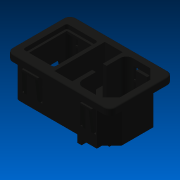
# Autodesk Inventor part: Soanar Power Module Housing
Saved by Autodesk Inventor 2016 (Build 200138000, 138)
## iProperties
Created: 2013-08-06
Material: ABS Plastic
Document SubType Name: Modeling
Designer: sdarley
Density: 1.06 g/cm^3
Appearance: Smooth - Black
Project: Power Entry Module - Soanar PP4003
Description: Soanar Power Module Housing
Author: sdarley
Title: Soanar Power Module Housing
Revision Number: 1
Autodesk Inventor part; units mm, degrees
ref_plane "YZ Plane" through (0, 0, 0) normal (1, 0, 0) x (0, 1, 0)
sketch "Sketch1" plane through (0, 0, 0) normal (0, 1, 0) x (-1, 0, 0)
  line L0 (-22, -15.3) -> (22, -15.3)
  line L1 (25, -12.3) -> (25, 12.3)
  line L2 (22, 15.3) -> (-22, 15.3)
  line L3 (-25, 12.3) -> (-25, -12.3)
  line L4 (-25, -15.3) -> (25, 15.3) construction
  line L5 (25, -15.3) -> (-25, 15.3) construction
  arc A0 (-22, 15.3) -> (-25, 12.3) centre (-22, 12.3) ccw
  arc A1 (-25, -12.3) -> (-22, -15.3) centre (-22, -12.3) ccw
  arc A2 (22, -15.3) -> (25, -12.3) centre (22, -12.3) ccw
  arc A3 (25, 12.3) -> (22, 15.3) centre (22, 12.3) ccw
  line L6 (20.8, 10.65) -> (7.8, 10.65)
  line L7 (6.8, 9.65) -> (6.8, -9.65)
  line L8 (7.8, -10.65) -> (20.8, -10.65)
  line L9 (21.8, -9.65) -> (21.8, 9.65)
  line L10 (5, 12.15) -> (-3.6, 12.15)
  line L11 (-3.6, -12.15) -> (5, -12.15)
  line L12 (5, -12.15) -> (5, 12.15)
  arc A4 (7.8, 10.65) -> (6.8, 9.65) centre (7.8, 9.65) ccw
  arc A5 (21.8, 9.65) -> (20.8, 10.65) centre (20.8, 9.65) ccw
  arc A6 (20.8, -10.65) -> (21.8, -9.65) centre (20.8, -9.65) ccw
  arc A7 (6.8, -9.65) -> (7.8, -10.65) centre (7.8, -9.65) ccw
  line L13 (-3.6, -2.55) -> (-5.45, -2.55)
  line L14 (-5.45, -2.55) -> (-5.45, -9.1)
  line L15 (-8.45, -12.1) -> (-16.95, -12.1)
  line L16 (-16.95, -12.1) -> (-21.8, -7.25)
  line L17 (-21.8, -7.25) -> (-21.8, 7.25)
  line L18 (-21.8, 7.25) -> (-16.95, 12.1)
  line L19 (-16.95, 12.1) -> (-8.45, 12.1)
  line L20 (-3.6, 2.55) -> (-5.45, 2.55)
  line L21 (-5.45, 2.55) -> (-5.45, 9.1)
  line L22 (-3.6, 12.15) -> (-3.6, 2.55)
  line L23 (-3.6, -2.55) -> (-3.6, -12.15)
  arc A8 (-8.45, -12.1) -> (-5.45, -9.1) centre (-8.45, -9.1) ccw
  arc A9 (-5.45, 9.1) -> (-8.45, 12.1) centre (-8.45, 9.1) ccw
  point P0 (0, 0)
  point P1 (0, 0)
  point P2 (6.8, 0)
  point P3 (5, 0)
  point P4 (0, 0)
  point P5 (-21.8, 0)
  dimension "d0" = 50
  dimension "d1" = 30.6
  dimension "d2" = 3
  dimension "d5" = 21.3
  dimension "d6" = 15
  dimension "d7" = 3.2
  dimension "d8" = 1
  dimension "d10" = 1.8
  dimension "d11" = 24.3
  dimension "d12" = 8.6
  dimension "d13" = 5.1
  dimension "d14" = 24.2
  dimension "d15" = 14.5
  dimension "d16" = 12.1
  dimension "d17" = 16.35
  dimension "d19" = 1.85
  dimension "d20" = 3
  constraints: 48 end point, 20 point on circle, 20 tangent, 10 centre point, 10 perpendicular, 9 parallel, 8 point on line, 7 equal radius, 7 midpoint, 3 horizontal, 3 horizontal alignment, 2 equal length, 2 vertical alignment
  measures "d0" distance of L5.end L4.end
  measures "d1" distance of L4.end L5.start
  measures "d2" radius of A0
  measures "d5" distance between parallel lines of L8 L6
  measures "d6" distance between parallel lines of L9 L7
  measures "d7" distance between parallel lines of L1 L9
  measures "d8" radius of A4
  measures "d10" distance between parallel lines of L12 L7
  measures "d11" distance between parallel lines of L10 L11
  measures "d12" distance between parallel lines of L12 L23
  measures "d13" distance between parallel lines of L20 L13
  measures "d14" distance between parallel lines of L19 L15
  measures "d15" distance of L16.end L17.end
  measures "d16" distance from line of point (0, 0) L15
  measures "d17" distance between parallel lines of L17 L14
  measures "d19" distance between parallel lines of L14 L23
  measures "d20" radius of A8
extrude "Extrusion1" add sketch "Sketch1" against normal blind 3.15
sketch "Sketch2" plane through (0, -3.15, 0) normal (0, -1, 0) x (1, 0, 0)
  arc A0 (-6.8, 9.65) -> (-7.8, 10.65) centre (-7.8, 9.65) ccw projected
  line L0 (-6.8, 9.65) -> (-6.8, -9.65) projected
  arc A1 (-7.8, -10.65) -> (-6.8, -9.65) centre (-7.8, -9.65) ccw projected
  line L1 (-7.8, -10.65) -> (-20.8, -10.65) projected
  arc A2 (-21.8, -9.65) -> (-20.8, -10.65) centre (-20.8, -9.65) ccw projected
  line L2 (-21.8, -9.65) -> (-21.8, 9.65) projected
  arc A3 (-20.8, 10.65) -> (-21.8, 9.65) centre (-20.8, 9.65) ccw projected
  line L3 (-20.8, 10.65) -> (-7.8, 10.65) projected
  line L4 (-20.75, 9.6) -> (-7.85, 9.6)
  line L5 (-7.85, 9.6) -> (-7.85, -9.6)
  line L6 (-7.85, -9.6) -> (-20.75, -9.6)
  line L7 (-20.75, -9.6) -> (-20.75, 9.6)
  point P0 (0, 0)
  point P1 (-14.3, 9.6)
  point P2 (-14.3, 10.65)
  point P3 (-20.75, 0)
  point P4 (-21.8, 0)
  dimension "d21" = 19.2
  dimension "d22" = 12.9
  constraints: 8 end point, 4 midpoint, 2 parallel, 1 horizontal, 1 horizontal alignment, 1 perpendicular, 1 vertical alignment
  measures "d21" distance between parallel lines of L6 L4
  measures "d22" distance between parallel lines of L5 L7
extrude "Extrusion2" add sketch "Sketch2" against normal blind 1.15
sketch "Sketch3" plane through (0, -3.15, 0) normal (0, -1, 0) x (1, 0, 0)
  line L0 (-20.75, -9.6) -> (-20.75, 9.6) projected
  line L1 (-20.75, 9.6) -> (-7.85, 9.6) projected
  line L2 (-7.85, 9.6) -> (-7.85, -9.6) projected
  line L3 (-7.85, -9.6) -> (-20.75, -9.6) projected
  line L4 (3.6, 12.15) -> (3.6, 2.55) projected
  line L5 (3.6, 2.55) -> (5.45, 2.55) projected
  line L6 (5.45, 2.55) -> (5.45, 9.1) projected
  arc A0 (8.45, 12.1) -> (5.45, 9.1) centre (8.45, 9.1) ccw projected
  line L7 (8.45, 12.1) -> (16.95, 12.1) projected
  line L8 (16.95, 12.1) -> (21.8, 7.25) projected
  line L9 (21.8, 7.25) -> (21.8, -7.25) projected
  line L10 (21.8, -7.25) -> (16.95, -12.1) projected
  line L11 (16.95, -12.1) -> (8.45, -12.1) projected
  arc A1 (5.45, -9.1) -> (8.45, -12.1) centre (8.45, -9.1) ccw projected
  line L12 (5.45, -9.1) -> (5.45, -2.55) projected
  line L13 (5.45, -2.55) -> (3.6, -2.55) projected
  line L14 (3.6, -2.55) -> (3.6, -12.15) projected
  line L15 (3.6, -12.15) -> (-5, -12.15) projected
  line L16 (-5, -12.15) -> (-5, 12.15) projected
  line L17 (-5, 12.15) -> (3.6, 12.15) projected
  line L18 (-22, -15.3) -> (22, -15.3) projected
  line L19 (-20.4, 13.6) -> (16.9, 13.6)
  line L20 (16.9, 13.6) -> (22.9, 7.6)
  line L21 (22.9, 7.6) -> (22.9, -7.6)
  line L22 (22.9, -7.6) -> (16.9, -13.6)
  line L23 (16.9, -13.6) -> (-20.4, -13.6)
  line L24 (-22.9, 11.1) -> (-22.9, -11.1)
  arc A2 (-20.4, 13.6) -> (-22.9, 11.1) centre (-20.4, 11.1) ccw
  arc A3 (-22.9, -11.1) -> (-20.4, -13.6) centre (-20.4, -11.1) ccw
  point P0 (0, 0)
  point P1 (-22.9, 0)
  point P2 (22.9, 0)
  dimension "d26" = 45.8
  dimension "d27" = 27.2
  dimension "d28" = 22.9
  dimension "d29" = 6
  dimension "d30" = 2.5
  constraints: 12 end point, 4 perpendicular, 4 point on circle, 4 tangent, 2 centre point, 2 horizontal alignment, 2 midpoint, 2 parallel, 1 equal radius
  measures "d26" distance between parallel lines of L21 L24
  measures "d27" distance between parallel lines of L23 L19
  measures "d28" distance from line of point (0, 0) L24
  measures "d29" horizontal distance of L20.end L19.end
  measures "d30" radius of A2
extrude "Extrusion3" add sketch "Sketch3" along normal blind 16.35
sketch "Sketch4" plane through (0, -19.5, 0) normal (0, -1, 0) x (1, 0, 0)
  line L0 (-20.75, 9.6) -> (-7.85, 9.6) projected
  line L1 (-7.85, 9.6) -> (-7.85, -9.6) projected
  line L2 (-7.85, -9.6) -> (-20.75, -9.6) projected
  line L3 (-20.75, -9.6) -> (-20.75, 9.6) projected
  line L4 (-19.575, 12.3) -> (-9.025, 12.3)
  line L5 (-6.525, 9.8) -> (-6.525, -9.8)
  line L6 (-9.025, -12.3) -> (-19.575, -12.3)
  line L7 (-22.075, -9.8) -> (-22.075, 9.8)
  arc A0 (-19.575, 12.3) -> (-22.075, 9.8) centre (-19.575, 9.8) ccw
  arc A1 (-6.525, 9.8) -> (-9.025, 12.3) centre (-9.025, 9.8) ccw
  arc A2 (-9.025, -12.3) -> (-6.525, -9.8) centre (-9.025, -9.8) ccw
  arc A3 (-22.075, -9.8) -> (-19.575, -12.3) centre (-19.575, -9.8) ccw
  point P0 (0, 0)
  point P1 (-14.3, 12.3)
  point P2 (-14.3, 9.6)
  point P3 (-22.075, 0)
  point P4 (-20.75, 0)
  dimension "d33" = 15.55
  dimension "d34" = 24.6
  dimension "d35" = 2.5
  constraints: 8 end point, 8 point on circle, 8 tangent, 4 centre point, 4 midpoint, 3 equal radius, 2 parallel, 1 horizontal, 1 horizontal alignment, 1 perpendicular, 1 vertical alignment
  measures "d33" distance between parallel lines of L5 L7
  measures "d34" distance between parallel lines of L6 L4
  measures "d35" radius of A0
extrude "Extrusion4" cut sketch "Sketch4" against normal blind 16.35
sketch "Sketch5" plane through (-22.9, -3.15, -11.1) normal (-1, 0, 0) x (0, 0, 1)
  line L0 (22.2, -16.35) -> (0, -16.35) projected
  line L1 (22.2, 0) -> (22.2, -16.35) projected
  line L2 (2.675, -16.35) -> (3.85, -10.5)
  line L3 (3.85, -10.5) -> (18.35, -10.5)
  line L4 (18.35, -10.5) -> (19.525, -16.35)
  line L5 (2.675, -16.35) -> (19.525, -16.35)
  point P0 (11.1, 3.15)
  point P1 (11.1, -10.5)
  point P2 (11.1, -16.35)
  dimension "d38" = 14.5
  dimension "d39" = 16.85
  dimension "d40" = 5.85
  constraints: 8 end point, 3 midpoint, 2 point on line, 1 collinear, 1 perpendicular, 1 vertical alignment
  measures "d38" distance of L2.end L3.end
  measures "d39" distance of L4.end L2.start
  measures "d40" distance between parallel lines of L3 L0
extrude "Extrusion5" cut sketch "Sketch5" against normal up to surface (0.825 mm away)
sketch "Sketch6" plane through (0, -19.5, 0) normal (0, -1, 0) x (1, 0, 0)
  line L0 (3.6, 2.55) -> (5.45, 2.55) projected
  line L1 (5.45, 2.55) -> (5.45, 9.1) projected
  arc A0 (8.45, 12.1) -> (5.45, 9.1) centre (8.45, 9.1) ccw projected
  line L2 (8.45, 12.1) -> (16.95, 12.1) projected
  line L3 (16.95, 12.1) -> (21.8, 7.25) projected
  line L4 (21.8, 7.25) -> (21.8, -7.25) projected
  line L5 (21.8, -7.25) -> (16.95, -12.1) projected
  line L6 (16.95, -12.1) -> (8.45, -12.1) projected
  arc A1 (5.45, -9.1) -> (8.45, -12.1) centre (8.45, -9.1) ccw projected
  line L7 (5.45, -9.1) -> (5.45, -2.55) projected
  line L8 (5.45, -2.55) -> (3.6, -2.55) projected
  line L9 (3.6, -2.55) -> (3.6, -12.15) projected
  line L10 (3.6, -12.15) -> (-5, -12.15) projected
  line L11 (-5, -12.15) -> (-5, 12.15) projected
  line L12 (-5, 12.15) -> (3.6, 12.15) projected
  line L13 (3.6, 12.15) -> (3.6, 2.55) projected
  circle A2 centre (-0.7, 0) radius 1.95
  point P0 (0, 0)
  point P1 (-0.7, 12.15)
  point P2 (-5, 0)
  dimension "d43" = 3.9
  constraints: 2 midpoint, 1 centre point, 1 horizontal alignment, 1 vertical alignment
  measures "d43" diameter of A2
extrude "Extrusion6" add sketch "Sketch6" against normal blind 1.75
sketch "Sketch7" plane through (0, -17.75, 0) normal (0, 1, 0) x (1, 0, 0)
  line L0 (5.45, -9.1) -> (5.45, -2.55) projected
  arc A0 (5.45, -9.1) -> (8.45, -12.1) centre (8.45, -9.1) ccw projected
  line L1 (16.95, -12.1) -> (8.45, -12.1) projected
  line L2 (21.8, -7.25) -> (16.95, -12.1) projected
  line L3 (21.8, 7.25) -> (21.8, -7.25) projected
  line L4 (16.95, 12.1) -> (21.8, 7.25) projected
  line L5 (8.45, 12.1) -> (16.95, 12.1) projected
  arc A1 (8.45, 12.1) -> (5.45, 9.1) centre (8.45, 9.1) ccw projected
  line L6 (5.45, 2.55) -> (5.45, 9.1) projected
  line L7 (3.6, -2.55) -> (3.6, -12.15) projected
  line L8 (5.45, 2.55) -> (7.75, 2.55)
  line L9 (7.75, 2.55) -> (7.75, -2.55)
  line L10 (7.75, -2.55) -> (5.45, -2.55)
  point P0 (0, 0)
  dimension "d46" = 2.3
  constraints: 6 end point, 2 perpendicular, 1 parallel
  measures "d46" distance between parallel lines of L9 L6
extrude "Extrusion7" add sketch "Sketch7" along normal blind 1.15
sketch "Sketch8" plane through (0, -17.75, 0) normal (0, 1, 0) x (1, 0, 0)
  line L0 (3.6, 2.55) -> (7.75, 2.55) projected
  line L1 (7.75, -2.55) -> (3.6, -2.55) projected
  line L2 (7.75, -2.55) -> (7.75, 2.55) projected
  line L3 (3.6, 2.55) -> (3.6, -2.55)
  point P0 (0, 0)
  constraints: 2 end point, 1 parallel
extrude "Extrusion8" cut sketch "Sketch8" against normal blind 0.85
sketch "Sketch9" plane through (0, -3.15, 0) normal (0, -1, 0) x (1, 0, 0)
  line L0 (16.9, 13.6) -> (22.9, 7.6) projected
  line L1 (22.9, -7.6) -> (16.9, -13.6) projected
  line L2 (-22, -15.3) -> (22, -15.3) projected
  line L3 (16.9, 13.6) -> (21.7, 13.6)
  line L4 (22.9, 12.4) -> (22.9, 7.6)
  line L5 (22.9, -7.6) -> (22.9, -12.4)
  line L6 (21.7, -13.6) -> (16.9, -13.6)
  arc A0 (22.9, 12.4) -> (21.7, 13.6) centre (21.7, 12.4) ccw
  arc A1 (21.7, -13.6) -> (22.9, -12.4) centre (21.7, -12.4) ccw
  point P0 (0, 0)
  dimension "d51" = 1.2
  constraints: 8 end point, 4 point on circle, 4 tangent, 2 centre point, 2 perpendicular, 1 collinear, 1 equal radius, 1 parallel
  measures "d51" radius of A0
extrude "Extrusion9" cut sketch "Sketch9" against normal blind 1.6
sketch "Sketch10" plane through (0, -19.5, 0) normal (0, -1, 0) x (1, 0, 0)
  line L0 (-20.4, -13.6) -> (16.9, -13.6) projected
  line L1 (22.9, 7.6) -> (16.9, 13.6) projected
  line L2 (16.9, 13.6) -> (-20.4, 13.6) projected
  line L3 (-22.9, 11.1) -> (-22.9, 8.425) projected
  line L4 (8.6, -13.6) -> (8.6, -11.1)
  line L5 (16.9, -13.6) -> (16.9, -4.7)
  line L6 (16.9, 13.6) -> (16.9, 4.7)
  line L7 (16.9, 4.7) -> (17.675, 4.7)
  line L8 (16.9, -4.7) -> (17.675, -4.7)
  line L9 (17.675, -3.05) -> (14, -3.05)
  line L10 (14, -3.05) -> (12.5, -1.55)
  line L11 (12.5, -1.55) -> (12.5, 1.55)
  line L12 (12.5, 1.55) -> (14, 3.05)
  line L13 (14, 3.05) -> (17.675, 3.05)
  arc A0 (17.675, 3.05) -> (17.675, 4.7) centre (17.675, 3.875) ccw
  arc A1 (17.675, -4.7) -> (17.675, -3.05) centre (17.675, -3.875) ccw
  line L14 (7.45, 13.6) -> (7.45, 11.1)
  line L15 (7.45, 11.1) -> (13.4, 11.1)
  line L16 (13.4, 11.1) -> (13.4, 10.1)
  line L17 (13.4, 10.1) -> (14.9, 8.6)
  line L18 (14.9, 8.6) -> (14.9, 5.2)
  line L19 (14.9, 5.2) -> (13.4, 3.7)
  line L20 (13.4, 3.7) -> (9.6375, 3.7)
  line L21 (9.6375, 2.125) -> (10.9, 2.125)
  line L22 (10.9, 2.125) -> (10.9, -2.125)
  line L23 (10.9, -2.125) -> (9.6375, -2.125)
  line L24 (9.6375, -3.7) -> (13.4, -3.7)
  line L25 (13.4, -3.7) -> (14.9, -5.2)
  line L26 (14.9, -5.2) -> (14.9, -8.6)
  line L27 (14.9, -8.6) -> (13.4, -10.1)
  line L28 (13.4, -10.1) -> (13.4, -11.1)
  line L29 (13.4, -11.1) -> (8.6, -11.1)
  arc A2 (9.6375, 3.7) -> (9.6375, 2.125) centre (9.6375, 2.9125) ccw
  arc A3 (9.6375, -2.125) -> (9.6375, -3.7) centre (9.6375, -2.9125) ccw
  point P0 (0, 0)
  point P1 (12.5, 0)
  point P2 (10.9, 0)
  dimension "d54" = 9.4
  dimension "d55" = 6.1
  dimension "d56" = 3.1
  dimension "d57" = 4.4
  dimension "d58" = 1.6
  dimension "d59" = 9.45
  dimension "d60" = 2.5
  dimension "d61" = 7.4
  dimension "d62" = 4.25
  dimension "d63" = 2.05
  dimension "d64" = 1.6
  dimension "d65" = 4.8
  dimension "d67" = 1
  dimension "d116" = 8.3
  dimension "d117" = 2
  constraints: 52 end point, 14 perpendicular, 9 parallel, 9 vertical alignment, 8 point on circle, 8 tangent, 4 centre point, 4 equal length, 2 equal radius, 2 horizontal alignment, 2 midpoint, 2 point on line, 1 collinear, 1 horizontal
  measures "d54" distance between parallel lines of L8 L7
  measures "d55" distance between parallel lines of L9 L13
  measures "d56" distance of L10.end L11.end
  measures "d57" distance between parallel lines of L6 L11
  measures "d59" distance between parallel lines of L14 L6
  measures "d60" distance between parallel lines of L0 L29
  measures "d61" distance between parallel lines of L29 L24
  measures "d62" distance between parallel lines of L23 L21
  measures "d64" distance between parallel lines of L11 L22
  measures "d65" distance of L28.end L4.end
  measures "d67" distance of L15.end L16.end
  measures "d116" distance between parallel lines of L5 L4
  measures "d117" distance between parallel lines of L5 L26
extrude "Extrusion10" add sketch "Sketch10" along normal blind 1.3
sketch "Sketch11" plane through (0, -20.8, 0) normal (0, -1, 0) x (1, 0, 0)
  line L0 (16.9, -13.6) -> (16.9, -4.7) projected
  line L1 (17.675, -3.05) -> (14, -3.05) projected
  line L2 (14, -3.05) -> (12.5, -1.55) projected
  line L3 (12.5, -1.55) -> (12.5, 1.55) projected
  line L4 (12.5, 1.55) -> (14, 3.05) projected
  line L5 (14, 3.05) -> (17.675, 3.05) projected
  line L6 (16.9, 4.7) -> (16.9, 13.6) projected
  line L7 (16.9, 13.6) -> (7.45, 13.6) projected
  line L8 (7.45, 13.6) -> (7.45, 11.1) projected
  line L9 (7.45, 11.1) -> (13.4, 11.1) projected
  line L10 (14.9, 8.6) -> (14.9, 5.2) projected
  line L11 (14.9, 5.2) -> (13.4, 3.7) projected
  line L12 (13.4, 3.7) -> (9.6375, 3.7) projected
  line L13 (9.6375, 2.125) -> (10.9, 2.125) projected
  line L14 (10.9, 2.125) -> (10.9, -2.125) projected
  line L15 (9.6375, -3.7) -> (13.4, -3.7) projected
  line L16 (13.4, -3.7) -> (14.9, -5.2) projected
  line L17 (14.9, -5.2) -> (14.9, -8.6) projected
  line L18 (8.6, -13.6) -> (16.9, -13.6) projected
  line L19 (9.55, 13.6) -> (9.55, 11.1)
  line L20 (14.9, 7.5) -> (16.9, 7.5)
  line L21 (10.9, 3.7) -> (10.9, 2.125)
  line L22 (10.9, -2.125) -> (10.9, -3.7)
  line L23 (16.9, 4.7) -> (16.9, 3.05)
  line L24 (16.9, -3.05) -> (16.9, -4.7)
  line L25 (14.9, -7.5) -> (16.9, -7.5)
  point P0 (0, 0)
  dimension "d70" = 2.1
  dimension "d71" = 15
  dimension "d72" = 7.5
  constraints: 14 end point, 10 point on line, 6 perpendicular, 1 collinear
  measures "d70" distance between parallel lines of L8 L19
  measures "d71" distance between parallel lines of L25 L20
  measures "d72" distance from line of point (0, 0) L20
extrude "Extrusion11" add sketch "Sketch11" along normal blind 2.25
sketch "Sketch22" plane through (0, -19.5, 0) normal (0, -1, 0) x (1, 0, 0)
  line L0 (-22.9, 11.1) -> (-22.9, 8.425) projected
  line L1 (-20.4, -13.6) -> (8.6, -13.6) projected
  line L2 (-4.95, 7.2) -> (3.4, 7.2)
  line L3 (3.9, 6.7) -> (3.9, 3.55)
  line L4 (3.4, 3.05) -> (-4.95, 3.05)
  line L5 (-5.45, 3.55) -> (-5.45, 6.7)
  arc A0 (-4.95, 7.2) -> (-5.45, 6.7) centre (-4.95, 6.7) ccw
  arc A1 (-5.45, 3.55) -> (-4.95, 3.05) centre (-4.95, 3.55) ccw
  arc A2 (3.4, 3.05) -> (3.9, 3.55) centre (3.4, 3.55) ccw
  arc A3 (3.9, 6.7) -> (3.4, 7.2) centre (3.4, 6.7) ccw
  point P0 (0, 0)
  point P1 (-5.45, 7.2)
  point P2 (3.9, 3.05)
  point P3 (3.9, 7.2)
  point P4 (-5.45, 3.05)
  dimension "d118" = 9.35
  dimension "d119" = 4.15
  dimension "d120" = 20.8
  dimension "d121" = 17.45
  dimension "d124" = 0.5
  constraints: 8 end point, 8 point on circle, 8 point on line, 8 tangent, 4 centre point, 3 equal radius, 2 parallel, 1 horizontal, 1 perpendicular
  measures "d118" distance of point (-5.45, 7.2) point (3.9, 7.2)
  measures "d119" distance between parallel lines of L4 L2
  measures "d120" distance between parallel lines of L1 L2
  measures "d121" distance between parallel lines of L0 L5
  measures "d124" radius of A0
extrude "Extrusion22" add sketch "Sketch22" along normal blind 0.3
ref_plane "Work Plane1" through (-14.3, -19.5, -9.8) normal (-1, 0, 0) x (0, 0, 1)
sketch "Sketch12" plane through (-14.3, -19.5, -9.8) normal (-1, 0, 0) x (0, 0, 1)
  line L0 (-2.5, 19.5) -> (-5.5, 19.5) projected
  line L1 (-2.5, 19.5) -> (-2.5, 16.35) projected
  line L2 (-5.5, 16.35) -> (-2.5, 16.35) projected
  line L3 (-5.5, 19.5) -> (-5.5, 16.35) projected
  line L4 (-2.5, 0) -> (-2.5, 16.35) projected
  line L5 (-3.8, 16.35) -> (-3.8, 0) projected
  line L6 (25.1, 19.5) -> (22.1, 19.5) projected
  line L7 (25.1, 19.5) -> (25.1, 16.35) projected
  line L8 (22.1, 16.35) -> (25.1, 16.35) projected
  line L9 (22.1, 19.5) -> (22.1, 16.35) projected
  line L10 (23.4, 16.35) -> (23.4, 0) projected
  line L11 (22.1, 0) -> (22.1, 16.35) projected
  line L12 (-3.8, 16.35) -> (-2.5, 16.35)
  line L13 (-2.5, 16.35) -> (-2.5, 15.05)
  line L14 (-2.5, 15.05) -> (-3.8, 15.05)
  line L15 (-3.8, 15.05) -> (-3.8, 16.35)
  line L16 (23.4, 16.35) -> (22.1, 16.35)
  line L17 (22.1, 16.35) -> (22.1, 15.05)
  line L18 (22.1, 15.05) -> (23.4, 15.05)
  line L19 (23.4, 15.05) -> (23.4, 16.35)
  point P0 (9.8, 19.5)
  dimension "d85" = 1.3
  constraints: 16 end point, 4 parallel, 2 horizontal, 2 perpendicular, 2 point on line, 1 horizontal alignment
  measures "d85" distance of L12.end L13.end
extrude "Extrusion12" cut sketch "Sketch12" along normal mid plane 9.8 contours L4 L14 L5 L2 | L8 L10 L18 L11
sketch "Sketch14" plane through (-9.4, -19.5, -9.8) normal (-1, 0, 0) x (0, 0, 1)
  line L0 (-3.8, 15.05) -> (-3.8, 16.35) projected
  line L1 (-2.5, 16.35) -> (-2.5, 15.05) projected
  line L2 (-3.8, 16.35) -> (-2.5, 16.35) projected
  line L3 (-3.8, 15.05) -> (-2.5, 15.05)
  line L4 (-2.5, 15.05) -> (-2.5, 4.35)
  line L5 (-2.5, 4.35) -> (-3.8, 4.35)
  line L6 (-3.8, 4.35) -> (-3.8, 15.05)
  line L7 (23.4, 15.05) -> (22.1, 15.05) projected
  line L8 (23.4, 16.35) -> (23.4, 15.05) projected
  line L9 (22.1, 16.35) -> (23.4, 16.35) projected
  line L10 (22.1, 15.05) -> (22.1, 16.35) projected
  line L11 (22.1, 15.05) -> (23.4, 15.05)
  line L12 (23.4, 15.05) -> (23.4, 4.35)
  line L13 (23.4, 4.35) -> (22.1, 4.35)
  line L14 (22.1, 4.35) -> (22.1, 15.05)
  point P0 (9.8, 19.5)
  dimension "d86" = 12
  constraints: 16 end point, 4 parallel, 2 horizontal, 2 perpendicular, 1 horizontal alignment, 1 point on line
  measures "d86" distance between parallel lines of L5 L2
extrude "Extrusion14" cut sketch "Sketch14" along normal blind 1 contours L0 L2 L1 L3 | L3 L4 L5 L6 | L12 L13 L14 L7
sketch "Sketch15" plane through (-10.4, -19.5, -9.8) normal (1, 0, 0) x (0, 0, -1)
  line L0 (-23.4, 4.35) -> (-23.4, 15.05) projected
  line L1 (2.5, 15.05) -> (3.8, 15.05) projected
  line L2 (2.5, 4.35) -> (2.5, 15.05) projected
  line L3 (3.8, 4.35) -> (2.5, 4.35) projected
  line L4 (3.8, 15.05) -> (3.8, 4.35) projected
  line L5 (-23.4, 15.05) -> (-24.6, 15.05)
  line L6 (-24.6, 15.05) -> (-24.6, 14)
  line L7 (-24.6, 14) -> (-23.4, 4.35)
  line L8 (3.8, 15.05) -> (5, 15.05)
  line L9 (5, 15.05) -> (5, 14)
  line L10 (5, 14) -> (3.8, 4.35)
  point P0 (-9.8, 19.5)
  dimension "d89" = 1.2
  dimension "d90" = 1.05
  constraints: 12 end point, 4 perpendicular, 2 equal length
  measures "d89" distance between parallel lines of L0 L6
  measures "d90" distance from line of L5 L6.end
extrude "Extrusion15" add sketch "Sketch15" against normal blind 1.3 contours L7 L6 L5 L0 | L8 L9 L10 L4
sketch "Sketch17" plane through (-10.4, -19.5, -9.8) normal (1, 0, 0) x (0, 0, -1)
  line L0 (-22.1, 15.05) -> (-22.1, 4.35) projected
  line L1 (-22.1, 4.35) -> (-23.4, 4.35) projected
  line L2 (2.5, 15.05) -> (5, 15.05) projected
  line L3 (2.5, 4.35) -> (2.5, 15.05) projected
  line L4 (3.8, 4.35) -> (2.5, 4.35) projected
  line L5 (3.8, 4.35) -> (5, 14) projected
  line L6 (5, 14) -> (5, 15.05) projected
  line L7 (-22.1, 10.85) -> (-22.6, 10.85)
  line L8 (-22.6, 10.85) -> (-22.6, 9.95)
  line L9 (-22.6, 9.95) -> (-22.1, 9.95)
  line L10 (-22.1, 9.95) -> (-22.1, 10.85)
  line L11 (2.5, 10.85) -> (3, 10.85)
  line L12 (3, 10.85) -> (3, 9.95)
  line L13 (3, 9.95) -> (2.5, 9.95)
  line L14 (2.5, 9.95) -> (2.5, 10.85)
  point P0 (-9.8, 19.5)
  dimension "d95" = 0.9
  dimension "d96" = 5.6
  dimension "d97" = 0.5
  constraints: 16 end point, 4 parallel, 2 equal length, 2 horizontal, 2 perpendicular, 2 point on line, 1 horizontal alignment
  measures "d95" distance between parallel lines of L9 L7
  measures "d96" distance between parallel lines of L1 L9
  measures "d97" distance between parallel lines of L10 L8
extrude "Extrusion17" add sketch "Sketch17" along normal up to surface (1 mm away) contours L0 L9 L8 L7 | L11 L12 L13 L3
mirror "Mirror1" about plane through (-14.3, -19.5, -9.8) normal (-1, 0, 0) of "Extrusion14", "Extrusion15", "Extrusion17"
sketch "Sketch16" plane through (-16.9, -15.15, 13.6) normal (1, 0, 0) x (0, 0, -1)
  line L0 (-1.2, 10.7) -> (0, 10.7) projected
  line L1 (-1.2, 9.65) -> (-1.2, 10.7) projected
  line L2 (0, 10.7) -> (0, 0) projected
  line L3 (27.2, 0) -> (27.2, 10.7) projected
  line L4 (28.4, 9.65) -> (27.2, 0) projected
  line L5 (28.4, 10.7) -> (28.4, 9.65) projected
  line L6 (27.2, 10.7) -> (28.4, 10.7) projected
  line L7 (28.4, 9.65) -> (27.2, 9.65)
  line L8 (-1.2, 9.65) -> (0, 9.65)
  point P0 (13.6, 15.15)
  constraints: 4 end point, 2 perpendicular, 2 point on line
extrude "Extrusion16" add sketch "Sketch16" along normal up to surface (5.2 mm away) contours L0 L2 L8 L1 | L3 L6 L5 L7
ref_plane "Work Plane2" through (12.75, 0, 12.3) normal (1, 0, 0) x (0, 0, -1)
sketch "Sketch13" plane through (12.75, 0, 12.3) normal (1, 0, 0) x (0, 0, -1)
  line L0 (0, 0) -> (-3, 0) projected
  line L1 (0, 0) -> (0, -3.15) projected
  line L2 (-3, -3.15) -> (0, -3.15) projected
  line L3 (-3, 0) -> (-3, -3.15) projected
  line L4 (27.6, 0) -> (24.6, 0) projected
  line L5 (27.6, 0) -> (27.6, -3.15) projected
  line L6 (24.6, -3.15) -> (27.6, -3.15) projected
  line L7 (24.6, 0) -> (24.6, -3.15) projected
  line L8 (0.2, 0) -> (0.2, -16.6) projected
  line L9 (-1.3, -3.15) -> (-1.3, -15.15) projected
  line L10 (25.9, -15.15) -> (25.9, -3.15) projected
  line L11 (24.4, 0) -> (24.4, -16.6) projected
  line L12 (-1.3, -3.15) -> (0.2, -3.15)
  line L13 (0.2, -3.15) -> (0.2, -4.45)
  line L14 (0.2, -4.45) -> (-1.3, -4.45)
  line L15 (-1.3, -4.45) -> (-1.3, -3.15)
  line L16 (25.9, -3.15) -> (24.4, -3.15)
  line L17 (24.4, -3.15) -> (24.4, -4.45)
  line L18 (24.4, -4.45) -> (25.9, -4.45)
  line L19 (25.9, -4.45) -> (25.9, -3.15)
  dimension "d100" = 1.3
  constraints: 16 end point, 4 parallel, 2 horizontal, 2 perpendicular, 2 point on line, 1 horizontal alignment
  measures "d100" distance of L12.end L13.end
extrude "Extrusion13" cut sketch "Sketch13" along normal mid plane 7.5 contours L12 L8 L14 L9 L2 | L6 L10 L18 L11 L16
sketch "Sketch18" plane through (9, 0, 12.3) normal (1, 0, 0) x (0, 0, -1)
  line L0 (-1.3, -3.15) -> (0.2, -3.15) projected
  line L1 (24.4, -3.15) -> (25.9, -3.15) projected
  line L2 (24.4, -4.45) -> (24.4, -3.15) projected
  line L3 (25.9, -4.45) -> (24.4, -4.45) projected
  line L4 (25.9, -3.15) -> (25.9, -4.45) projected
  line L5 (-1.3, -4.45) -> (0.2, -4.45)
  line L6 (0.2, -4.45) -> (0.2, -15.15)
  line L7 (0.2, -15.15) -> (-1.3, -15.15)
  line L8 (-1.3, -15.15) -> (-1.3, -4.45)
  line L9 (25.9, -4.45) -> (24.4, -4.45)
  line L10 (24.4, -4.45) -> (24.4, -15.15)
  line L11 (24.4, -15.15) -> (25.9, -15.15)
  line L12 (25.9, -15.15) -> (25.9, -4.45)
  point P0 (12.3, 0)
  dimension "d101" = 12
  constraints: 16 end point, 4 parallel, 2 horizontal, 2 perpendicular, 1 horizontal alignment
  measures "d101" distance between parallel lines of L0 L7
extrude "Extrusion18" cut sketch "Sketch18" along normal blind 1 contours L3 L12 L11 L10 | L5 L6 L7 L8
sketch "Sketch19" plane through (10, 0, 12.3) normal (-1, 0, 0) x (0, 0, 1)
  line L0 (1.3, -4.45) -> (1.3, -15.15) projected
  line L1 (-24.4, -4.45) -> (-24.4, -15.15) projected
  line L2 (-25.9, -4.45) -> (-24.4, -4.45) projected
  line L3 (-25.9, -15.15) -> (-25.9, -4.45) projected
  line L4 (-24.4, -15.15) -> (-25.9, -15.15) projected
  line L5 (-25.9, -4.45) -> (-27.1, -4.45)
  line L6 (-27.1, -4.45) -> (-27.1, -5.5)
  line L7 (-27.1, -5.5) -> (-25.9, -15.15)
  line L8 (1.3, -4.45) -> (2.5, -4.45)
  line L9 (2.5, -4.45) -> (2.5, -5.5)
  line L10 (2.5, -5.5) -> (1.3, -15.15)
  point P0 (-12.3, 0)
  dimension "d104" = 1.05
  dimension "d105" = 1.2
  constraints: 12 end point, 3 perpendicular, 1 collinear, 1 horizontal alignment, 1 parallel
  measures "d104" distance from line of L6.end L5
  measures "d105" distance between parallel lines of L3 L6
extrude "Extrusion19" add sketch "Sketch19" against normal blind 1.3 contours L8 L9 L10 L0 | L3 L7 L6 L5
sketch "Sketch20" plane through (10, 0, 12.3) normal (-1, 0, 0) x (0, 0, 1)
  line L0 (-0.2, -15.15) -> (-0.2, -4.45) projected
  line L1 (-24.4, -4.45) -> (-24.4, -15.15) projected
  line L2 (-27.1, -4.45) -> (-24.4, -4.45) projected
  line L3 (-27.1, -4.45) -> (-27.1, -5.5) projected
  line L4 (-27.1, -5.5) -> (-25.9, -15.15) projected
  line L5 (-24.4, -15.15) -> (-25.9, -15.15) projected
  line L6 (-24.4, -8.65) -> (-24.9, -8.65)
  line L7 (-24.9, -8.65) -> (-24.9, -9.55)
  line L8 (-24.9, -9.55) -> (-24.4, -9.55)
  line L9 (-24.4, -9.55) -> (-24.4, -8.65)
  line L10 (-0.2, -8.65) -> (0.3, -8.65)
  line L11 (0.3, -8.65) -> (0.3, -9.55)
  line L12 (0.3, -9.55) -> (-0.2, -9.55)
  line L13 (-0.2, -9.55) -> (-0.2, -8.65)
  point P0 (-12.3, 0)
  dimension "d108" = 5.6
  dimension "d109" = 0.5
  dimension "d110" = 0.9
  constraints: 16 end point, 4 parallel, 2 equal length, 2 horizontal, 2 perpendicular, 2 point on line, 1 horizontal alignment
  measures "d108" distance between parallel lines of L8 L5
  measures "d109" distance between parallel lines of L1 L7
  measures "d110" distance between parallel lines of L6 L8
extrude "Extrusion20" add sketch "Sketch20" along normal up to surface (1 mm away) contours L0 L10 L11 L12 | L1 L8 L7 L6
mirror "Mirror2" about plane through (12.75, 0, 12.3) normal (1, 0, 0) of "Extrusion18", "Extrusion19", "Extrusion20"
sketch "Sketch21" plane through (14.2, -15.15, 13.6) normal (-1, 0, 0) x (0, 0, 1)
  line L0 (1.2, 10.7) -> (1.2, 9.65) projected
  line L1 (0, 10.7) -> (1.2, 10.7) projected
  line L2 (0, 0) -> (0, 10.7) projected
  line L3 (-28.4, 10.7) -> (-27.2, 10.7) projected
  line L4 (-28.4, 9.65) -> (-28.4, 10.7) projected
  line L5 (-27.2, 0) -> (-28.4, 9.65) projected
  line L6 (-27.2, 10.7) -> (-27.2, 0) projected
  line L7 (-28.4, 9.65) -> (-27.2, 9.65)
  line L8 (1.2, 9.65) -> (0, 9.65)
  point P0 (-13.6, 15.15)
  constraints: 4 end point, 2 point on line, 1 collinear, 1 perpendicular
extrude "Extrusion21" add sketch "Sketch21" along normal up to surface (2.9 mm away) contours L0 L8 L2 L1 | L3 L6 L7 L4
fillet "Fillet1" radius 0.5 8 edges at (24.1213, 0, 14.4213) (25, 0, 0) (24.1213, 0, -14.4213) (0, 0, -15.3) (-24.1213, 0, -14.4213) (-25, 0, 0) (-24.1213, 0, 14.4213) (0, 0, 15.3)
fillet "Fillet2" radius 5 8 edges at (-11.05, -5.5, 14.8) (-17.55, -5.5, 14.8) (10.65, -5.5, 14.8) (14.85, -5.5, 14.8) (14.85, -5.5, -14.8) (10.65, -5.5, -14.8) (-11.05, -5.5, -14.8) (-17.55, -5.5, -14.8)
equation "\"d16\" = 0.5 * d14"
equation "\"d28\" = 0.5 * d26"
equation "\"d72\" = 0.5 * d71"
body "Solid1"
